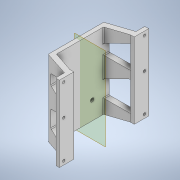
# Autodesk Inventor part: PiSpotAttachment
Saved by Autodesk Inventor 2021 (Build 250183000, 183)
## iProperties
Created: 2021-02-20
Part Number: PiSpotAttachment
Material: Generic
Document SubType Name: Modeling
Designer: mu3dp
Density: 1 g/cm^3
Appearance: Default
Author: mu3dp
Autodesk Inventor part; units mm, degrees
ref_plane "YZ Plane" through (0, 0, 0) normal (1, 0, 0) x (0, 1, 0)
ref_plane "XZ Plane" through (0, 0, 0) normal (0, 1, 0) x (-1, 0, 0)
ref_plane "XY Plane" through (0, 0, 0) normal (0, 0, 1) x (1, 0, 0)
sketch "Sketch1" plane through (0, 0, 0) normal (0, 1, 0) x (-1, 0, 0)
  line L0 (0, 96.3881) -> (0, -80.6119)
  line L1 (0, -80.6119) -> (7.6619, -80.6119)
  line L2 (7.6619, -80.6119) -> (7.6619, -63.0119)
  line L3 (7.6619, -63.0119) -> (55.6286, -47.1119)
  line L4 (55.6286, -47.1119) -> (55.6286, 62.8881)
  line L5 (55.6286, 62.8881) -> (7.6619, 78.7881)
  line L6 (7.6619, 78.7881) -> (7.6619, 96.3881)
  line L7 (7.6619, 96.3881) -> (0, 96.3881)
  point P0 (0, 0)
  dimension "d0" = 177
  dimension "d1" = 17.6
  dimension "d2" = 17.6
  dimension "d3" = 110
  dimension "d4" = 15.9
  constraints: 16 end point, 3 perpendicular, 2 point on line, 1 parallel
  measures "d0" distance of L0.start L0.end
  measures "d1" distance of L5.end L6.end
  measures "d2" distance of L1.end L2.end
  measures "d3" distance of L3.end L4.end
  measures "d4" vertical distance of L5.end L4.end
extrude "Extrusion1" add sketch "Sketch1" along normal blind 150
sketch "Sketch2" plane through (0, 150, 0) normal (0, 1, 0) x (1, 0, 0)
  line L0 (-7.6619, -78.7881) -> (-7.6619, -96.3881) projected
  line L1 (-7.6619, -78.7881) -> (0, -78.7881)
  line L2 (0, -96.3881) -> (0, 80.6119) projected
  line L3 (0, -78.7881) -> (0, -67.7881)
  line L4 (0, -67.7881) -> (-7.6619, -67.7881)
  line L5 (-7.6619, 80.6119) -> (-7.6619, 63.0119) projected
  line L6 (-7.6619, 63.0119) -> (0, 63.0119)
  line L7 (0, 63.0119) -> (0, 52.0119)
  line L8 (0, 52.0119) -> (-7.6619, 52.0119)
  line L9 (0, -67.7881) -> (0, 52.0119)
  line L10 (-7.6619, -67.7881) -> (-47.625, -54.5411)
  line L11 (-7.6619, 52.0119) -> (-47.625, 38.7649)
  line L12 (-55.6286, -62.8881) -> (-7.6619, -78.7881) projected
  line L13 (-7.6619, 63.0119) -> (-55.6286, 47.1119) projected
  line L14 (-47.625, -54.5411) -> (-47.625, 38.7649)
  point P0 (0, 0)
  dimension "d8" = 11
  dimension "d9" = 11
  dimension "d10" = 0
  dimension "d11" = 0
  dimension "d12" = 93.306
  constraints: 20 end point, 4 point on line, 3 perpendicular, 1 collinear, 1 horizontal, 1 vertical
  measures "d8" distance of L1.end L3.end
  measures "d9" distance of L6.end L7.end
  measures "d10" angle of L12 L10
  measures "d11" angle of L13 L11
  measures "d12" distance of L10.end L11.end
extrude "Extrusion2" cut sketch "Sketch2" against normal blind 150
sketch "Sketch3" plane through (0, 0, -80.6119) normal (0, 0, -1) x (-1, 0, 0)
  line L0 (0, 0) -> (0, 150) projected
  line L1 (0, 135) -> (7.7027, 135)
  line L2 (7.7027, 135) -> (47.625, 122.3)
  line L3 (47.625, 150) -> (47.625, 0) projected
  line L4 (47.625, 122.3) -> (47.625, 101.6779)
  line L5 (47.625, 101.6779) -> (7.6619, 88.9625)
  line L6 (7.6619, 150) -> (7.6619, 0) projected
  line L7 (7.6619, 88.9625) -> (0, 88.9625)
  line L8 (0, 135) -> (0, 88.9625)
  line L9 (0, 73.9625) -> (7.7027, 73.9625)
  line L10 (7.7027, 73.9625) -> (47.625, 61.2625)
  line L11 (47.625, 61.2625) -> (47.625, 27.7154)
  line L12 (47.625, 27.7154) -> (7.6619, 15)
  line L13 (7.6619, 15) -> (0, 15)
  line L14 (0, 73.9625) -> (0, 15)
  line L15 (0, 150) -> (7.6619, 150) projected
  line L16 (0, 0) -> (7.6619, 0) projected
  point P0 (7.6619, 15)
  point P1 (7.6619, 73.9625)
  point P2 (7.6619, 135)
  dimension "d15" = 72.35
  dimension "d16" = 72.353
  dimension "d18" = 15
  dimension "d19" = 15
  dimension "d20" = 46.0375
  dimension "d22" = 72.353
  dimension "d23" = 72.35
  dimension "d24" = 15
  constraints: 24 end point, 4 point on line, 2 horizontal, 1 collinear, 1 perpendicular
  measures "d15" angle of L5 L6
  measures "d16" angle of L6 L2
  measures "d18" distance between parallel lines of L9 L7
  measures "d19" distance between parallel lines of L15 L1
  measures "d20" distance between parallel lines of L1 L7
  measures "d22" angle of L6 L10
  measures "d23" angle of L6 L12
  measures "d24" distance between parallel lines of L16 L13
extrude "Extrusion3" cut sketch "Sketch3" against normal blind 1500 contours L6 L9 L10 L3 L12 | L6 L1 L2 L3 L5
fillet "Fillet1" radius 2 8 edges at (-47.625, 122.3, -44.2649) (-47.625, 101.6779, -44.2649) (-47.625, 61.2625, -44.2649) (-47.625, 27.7154, -44.2649) (-47.625, 61.2625, 60.0411) (-47.625, 122.3, 60.0411) (-47.625, 101.6779, 60.0411) (-47.625, 27.7154, 60.0411)
fillet "Fillet2" radius 2 12 edges at (-47.625, 121.5687, 54.5411) (-47.625, 136.15, 54.5411) (-47.625, 60.5312, 54.5411) (-47.625, 102.4092, 54.5411) (-47.625, 28.4467, 54.5411) (-47.625, 13.8577, 54.5411) (-47.625, 136.15, -38.7649) (-47.625, 121.5687, -38.7649) (-47.625, 60.5312, -38.7649) (-47.625, 102.4092, -38.7649) (-47.625, 13.8577, -38.7649) (-47.625, 28.4467, -38.7649)
fillet "Fillet3" radius 2 4 edges at (-7.6619, 75, 96.3881) (-7.6619, 75, -80.6119) (-55.6286, 75, -47.1119) (-55.6286, 75, 62.8881)
sketch "Sketch4" plane through (-7.6619, 15, -52.0119) normal (-1, 0, 0) x (0, 0, 1)
  line L0 (130.8, 135) -> (146.4, 135) projected
  line L1 (139.9, 135) -> (139.9, -14.5366)
  line L2 (-20.1, 135) -> (-20.1, -15)
  line L3 (-26.6, -15) -> (-26.6, 135) projected
  line L4 (-26.6, -15) -> (-11, -15) projected
  line L5 (148.4, -15) -> (148.4, 135) projected
  circle A0 centre (-20.1, 127.5) radius 2.475
  line L6 (-26.6, 135) -> (-11, 135) projected
  circle A1 centre (-20.1, 66.4625) radius 2.475
  circle A2 centre (-20.1, -7.5) radius 2.475
  line L7 (-10.9865, 58.9625) -> (0.0135, 58.9625) projected
  point P0 (52.0119, -15)
  dimension "d30" = 160
  dimension "d31" = 150
  dimension "d32" = 0
  dimension "d33" = 8.5
  dimension "d34" = 4.95
  dimension "d35" = 7.5
  dimension "d36" = 7.5
  dimension "d37" = 7.5
  constraints: 4 end point, 4 point on line, 3 centre point, 1 parallel, 1 vertical
  measures "d30" distance between parallel lines of L2 L1
  measures "d31" distance of L2.start L2.end
  measures "d32" distance from line of L4 L2.end
  measures "d33" distance between parallel lines of L5 L1
  measures "d34" diameter of A0
  measures "d35" distance from line of L6 A0.centre
  measures "d36" distance from line of A2.centre L4
  measures "d37" distance from line of L7 A1.centre
extrude "Extrusion4" cut sketch "Sketch4" against normal blind 1500 contours A0 L2 | L2 A0 | A1 L2 | L2 A1 | A2 L2 | L2 A2
ref_plane "Work Plane1" through (-221.551, 135, 7.8881) normal (0, 0, -1) x (0, -1, 0)
mirror "Mirror1" about plane through (-221.551, 135, 7.8881) normal (0, 0, -1) of "Extrusion4"
sketch "Sketch5" plane through (-55.6286, 0, -45.6678) normal (-1, 0, 0) x (0, 0, 1)
  line L0 (99.426, 7.686) -> (7.686, 7.686)
  line L1 (7.686, 7.686) -> (7.686, 65.906)
  line L2 (7.686, 65.906) -> (99.426, 65.906)
  line L3 (99.426, 65.906) -> (99.426, 7.686)
  line L4 (0, 0) -> (0, 150) projected
  line L5 (0, 0) -> (107.1119, 0) projected
  circle A0 centre (29.446, 35.966) radius 3.5498
  circle A1 centre (84.636, 35.966) radius 3.8886
  point P0 (45.6678, 0)
  dimension "d40" = 58.22
  dimension "d41" = 91.74
  dimension "d42" = 7.686
  dimension "d43" = 7.686
  dimension "d44" = 21.76
  dimension "d45" = 29.94
  dimension "d46" = 55.19
  dimension "d47" = 29.94
  constraints: 8 end point, 2 centre point, 2 parallel, 1 horizontal, 1 perpendicular
  measures "d40" distance between parallel lines of L2 L0
  measures "d41" distance of L0.start L0.end
  measures "d42" distance between parallel lines of L4 L1
  measures "d43" distance between parallel lines of L5 L0
  measures "d44" distance from line of L1 A0.centre
  measures "d45" distance from line of L2 A0.centre
  measures "d46" distance of A1.centre A0.centre
  measures "d47" distance from line of L2 A1.centre
extrude "Extrusion5" cut sketch "Sketch5" against normal blind 21.76 contours A0 | A1
equation "\"d48\" = d44"
body "Solid1"
